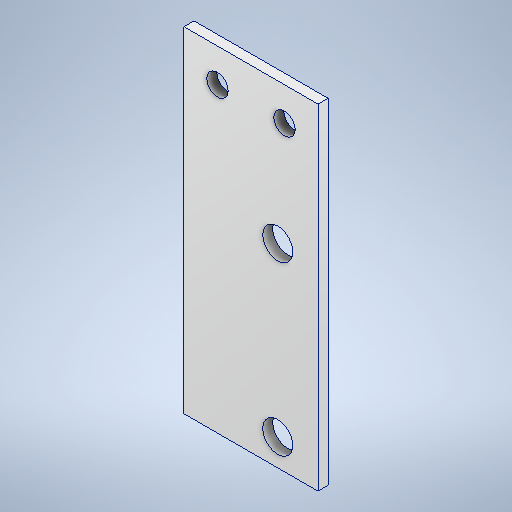
# Autodesk Inventor part: y_anchor_holder
Saved by Autodesk Inventor 2025 (Build 290162000, 162)
## iProperties
Created: 2024-04-25
Part Number: y_anchor_holder
Material: Hliník 6061
Document SubType Name: Modeling
Designer: rader
Density: 2.7 g/cm^3
Appearance: Hliník – plochý
Author: rader
Autodesk Inventor part; units mm, degrees
ref_plane "YZ Plane" through (0, 0, 0) normal (1, 0, 0) x (0, 1, 0)
ref_plane "XZ Plane" through (0, 0, 0) normal (0, 1, 0) x (-1, 0, 0)
ref_plane "XY Plane" through (0, 0, 0) normal (0, 0, 1) x (1, 0, 0)
sketch "Náčrt1" plane through (0, 0, 0) normal (0, 1, 0) x (-1, 0, 0)
  line L0 (10, 25) -> (-10, 25)
  line L1 (-10, 25) -> (-10, -25)
  line L2 (-10, -25) -> (10, -25)
  line L3 (10, -25) -> (10, 25)
  line L4 (0, -35) -> (0, 35) projected
  line L5 (-14, 0) -> (14, 0) projected
  point P0 (0, 0)
  dimension "d0" = 50
  dimension "d1" = 20
  constraints: 8 end point, 2 parallel, 1 horizontal, 1 perpendicular, 2 other
  measures "d0" distance of L0.end L1.end
  measures "d1" distance of L1.end L2.end
extrude "Vysunutí1" add sketch "Náčrt1" along normal mid plane 1.5
sketch "Náčrt2" plane through (0, 0.75, 0) normal (0, 1, 0) x (1, 0, 0)
  line L0 (-10, -25) -> (10, -25) projected
  line L1 (10, -25) -> (10, 25) projected
  line L2 (10, 25) -> (-10, 25) projected
  point P0 (0, 0)
  point P1 (5, -20)
  point P2 (-5, -20)
  dimension "d4" = 5
  dimension "d5" = 5
  dimension "d6" = 10
  dimension "d7" = 5
  measures "d4" distance from line of L0 point (-5, -20)
  measures "d5" distance from line of L0 point (5, -20)
  measures "d6" distance of point (5, -20) point (-5, -20)
  measures "d7" distance from line of L1 point (5, -20)
hole "Díra1" at (5, 0.75, 20) at (-5, 0.75, 20) direction (0, -1, 0) diameter 3.2 end through all
sketch "Náčrt3" plane through (0, 0.75, 0) normal (0, 1, 0) x (1, 0, 0)
  circle A0 centre (-5, -20) radius 1.6 projected
  circle A1 centre (5, -20) radius 1.6 projected
  line L0 (10, -25) -> (10, 25) projected
  line L1 (10, 25) -> (-10, 25) projected
  line L2 (-10, 25) -> (-10, -25) projected
  line L3 (-10, -25) -> (10, -25) projected
  point P0 (0, 0)
  point P1 (4, -4)
  point P2 (4, 21)
  dimension "d19" = 4
  dimension "d20" = 6
  dimension "d21" = 6
  dimension "d22" = 25
  measures "d19" distance from line of L1 point (4, 21)
  measures "d20" distance from line of L0 point (4, 21)
  measures "d21" distance from line of L0 point (4, -4)
  measures "d22" distance of point (4, 21) point (4, -4)
hole "Díra2" at (4, 0.75, 4) at (4, 0.75, -21) direction (0, -1, 0) diameter 4.5 end through all
